Autodesk Inventor part; units mm, degrees
(part 2 of 2)
sketch "Náčrt39" plane through (0, 0, 15.5) normal (0, -1, 0) x (1, 0, 0)
  line L0 (-46, 13.2) -> (-46, 26.7)
  line L1 (-33, 26.7) -> (-46, 26.7)
  line L2 (-33, 26.7) -> (-33, 13.2)
  line L3 (-46, 13.2) -> (-33, 13.2)
  line L4 (-21.25, 15.889) -> (-21.25, 29.639)
  line L5 (-11.5, 29.639) -> (-21.25, 29.639)
  line L6 (-11.5, 29.639) -> (-11.5, 30.839)
  line L7 (-8.5, 30.839) -> (-11.5, 30.839)
  line L8 (-8.5, 29.639) -> (-8.5, 30.839)
  line L9 (-8.5, 29.639) -> (-8.5, 15.889)
  line L10 (-8.5, 15.889) -> (-21.25, 15.889)
  line L11 (0, 30.082064) -> (0, 0)
  line L12 (0, 30.082064) -> (-2, 30.082064)
  line L13 (-2, 30.082064) -> (-2, 24.139)
  line L14 (-2, 24.139) -> (-4.75, 24.139)
  line L15 (-4.75, 24.139) -> (-4.75, 30.082064)
  line L16 (-4.75, 30.082064) -> (-22.45, 30.082064)
  line L17 (-22.45, 18.2) -> (-22.45, 30.082064)
  line L18 (-22.45, 18.2) -> (-32.2, 18.2)
  line L19 (-32.2, 27.9) -> (-32.2, 18.2)
  line L20 (-32.2, 27.9) -> (-46.8, 27.9)
  line L21 (-46.8, 27.9) -> (-46.8, 9.2)
  line L22 (-49.5, 9.2) -> (-46.8, 9.2)
  line L23 (-49.5, 0) -> (-49.5, 9.2)
  line L24 (-40.88345, 0) -> (-49.5, 0)
  line L25 (-40.88345, 0) -> (-40.88345, -5)
  line L26 (-36.02558, -5) -> (-40.88345, -5)
  line L27 (-36.02558, 0) -> (-36.02558, -5)
  line L28 (0, 0) -> (-36.02558, 0)
  line L29 (-2.5, 4.1) -> (-2.5, 14.689)
  line L30 (-2.5, 4.1) -> (-21.25, 4.1)
  line L31 (-21.25, 14.689) -> (-21.25, 4.1)
  line L32 (-2.5, 14.689) -> (-21.25, 14.689)
  line L33 (-46, 13.2) -> (-46, 26.7)
  line L34 (-46, 26.7) -> (-46, 27.9)
  line L35 (-32.2, 27.9) -> (-46.8, 27.9)
  line L36 (-45.6, 27.9) -> (-45.6, 21.7)
  line L37 (-45.6, 21.7) -> (-46, 21.7)
  line L38 (-33, 26.7) -> (-33, 27.9)
  line L39 (-33.4, 27.9) -> (-33.4, 21.7)
  line L40 (-33.4, 21.7) -> (-33, 21.7)
  line L41 (-21.25, 24.639) -> (-20.85, 24.639)
  line L42 (-20.85, 24.639) -> (-20.85, 30.839)
  line L43 (-21.25, 30.839) -> (-21.25, 29.639)
  line L44 (-8.9, 30.839) -> (-8.9, 24.639)
  line L45 (-8.9, 24.639) -> (-8.5, 24.639)
  line L46 (-8.5, 30.839) -> (-22.45, 30.839)
  point P0 (0, -15.5)
  point P1 (-21.45, 29.639)
  point P2 (-20.85, 29.639)
  point P3 (-21.45, 29.639)
  dimension "d1" = 2
  dimension "d347" = 0.4
  dimension "d348" = 5
  constraints: 22 end point, 13 point on line, 8 perpendicular, 5 equal length, 1 horizontal, 1 vertical
  measures "d347" distance between parallel lines of L0 L36
  measures "d348" distance between parallel lines of L37 L1
extrude "Vysunutí57" cut sketch "Náčrt39" against normal up to next contours L0 L1 L36 L37 | L34 L20 L36 L1 | L40 L39 L1 L2 | L1 L39 L20 L38 | L43 L46 L42 L16 | L16 L42 L5 L43 | L5 L42 L41 L4 | L44 L7 L8 L16 | L16 L8 L9 L45 L44
sketch "Náčrt40" plane through (-2.5, 0, 0) normal (-1, 0, 0) x (0, 0, 1)
  arc A0 (19.6, 15.5) -> (19.590814, 16.1) centre (0, 15.5) ccw
  arc A1 (19.590814, 16.1) -> (19.391686, 18.35) centre (0, 15.5) ccw
  arc A2 (19.391686, 18.35) -> (18.626594, 21.6) centre (0, 15.5) ccw
  arc A3 (18.626594, 21.6) -> (16.295147, 26.391657) centre (0, 15.5) ccw
  arc A4 (18.594508, 21.697118) -> (16.295147, 26.391657) centre (0, 15.5) ccw
  arc A5 (14.149289, 29.063098) -> (13.25, 29.942905) centre (0, 15.5) ccw
  arc A6 (13.25, 29.942905) -> (7.756288, 33.5) centre (0, 15.5) ccw
  arc A7 (19.6, 15.5) -> (7.756288, 33.5) centre (0, 15.5) ccw
  line L0 (7.193747, 33.5) -> (7.756288, 33.5)
  line L1 (13.25, 33.5) -> (7.756288, 33.5)
  line L2 (7.193747, 33.5) -> (13.25, 33.5)
  line L3 (7.193747, 33.5) -> (7.756288, 33.5)
  line L4 (7.193747, 33.5) -> (5.792097, 33.5)
  line L5 (5.792097, 33.5) -> (5.792097, 33.450985)
  line L6 (7.756288, 33.450985) -> (5.792097, 33.450985)
  line L7 (7.756288, 33.5) -> (7.756288, 33.450985)
  ellipse E0 centre (5.792097, 32.402567) end of major axis (6.890446, 32.402567) minor radius 1.097433 (5.792097, 33.5) -> (4.693747, 32.402567) ccw
  line L8 (4.693747, 32.402567) -> (4.693747, 32.353552)
  ellipse E1 centre (5.792097, 32.353552) end of major axis (6.890446, 32.353552) minor radius 1.097433 (5.792097, 33.450985) -> (4.693747, 32.353552) ccw
  line L9 (5.792097, 33.5) -> (5.792097, 33.450985)
  line L10 (4.693747, 32.402567) -> (4.693747, 29.75313)
  line L11 (4.693747, 29.75313) -> (4.693747, 29.704115)
  line L12 (4.693747, 32.353552) -> (4.693747, 29.704115)
  line L13 (4.693747, 32.402567) -> (4.693747, 32.353552)
  ellipse E2 centre (8.443747, 29.75313) end of major axis (12.193747, 29.75313) minor radius 3.74687 (4.693747, 29.75313) -> (6.568747, 26.508244) ccw
  line L14 (6.568747, 26.508244) -> (6.568747, 26.45923)
  ellipse E3 centre (8.443747, 29.704115) end of major axis (12.193747, 29.704115) minor radius 3.74687 (4.693747, 29.704115) -> (6.568747, 26.45923) ccw
  line L15 (4.693747, 29.75313) -> (4.693747, 29.704115)
  line L16 (6.568747, 26.508244) -> (15.5, 21.356087)
  line L17 (15.5, 21.356087) -> (15.5, 21.307072)
  line L18 (6.568747, 26.45923) -> (15.5, 21.307072)
  line L19 (6.568747, 26.508244) -> (6.568747, 26.45923)
  line L20 (5.193747, 28.839806) -> (5.193747, 32.353552)
  arc A8 (5.590195, 32.75) -> (5.193747, 32.353552) centre (5.590195, 32.353552) ccw
  line L21 (5.590195, 32.75) -> (9.305778, 32.75)
  arc A9 (5.193747, 28.839806) -> (6.568747, 26.45923) centre (7.942027, 28.839806) ccw
  point P0 (0, 0)
  point P1 (9.305778, 32.75)
  point P2 (7.756288, 33.5)
extrude "Vysunutí58" cut sketch "Náčrt40" along normal through all contours L21 A8 L20 A9 E2 L11 L10 L8 E1 L6 L7 A6 | L7 L6 L5 L4 L0 | L5 E1 E0 | A9 E3 E2
sketch "Náčrt41" plane through (0, 32, 7.193747) normal (0, 0, -1) x (-1, 0, 0)
  line L0 (0, 1.5) -> (2.5, 1.5) projected
  line L1 (0, 1.5) -> (0, 3.5)
  line L2 (0, 3.5) -> (1, 3.5)
  line L3 (1, 3.5) -> (1, 2)
  line L4 (1, 2) -> (2, 2)
  line L5 (2, 2) -> (2, 1.5)
  line L6 (2, 2) -> (2.5, 1.5)
  point P0 (0, -32)
  dimension "d357" = 1
  dimension "d358" = 0.5
  dimension "d359" = 2
  dimension "d360" = 1
  constraints: 12 end point, 3 perpendicular, 1 horizontal, 1 point on line, 1 vertical
  measures "d357" distance of L1.end L2.end
  measures "d358" distance from line of L3.end L0
  measures "d359" distance between parallel lines of L0 L2
  measures "d360" distance of L3.end L4.end
extrude "Vysunutí59" add sketch "Náčrt41" against normal up to surface (6.056253 mm away)
sketch "Náčrt42" plane through (-46.8, 2.241154, 16.5) normal (-1, 0, 0) x (0, 0, 1)
  line L0 (20.7, -1.041154) -> (12.2, -1.041154)
  line L1 (12.2, -1.041154) -> (20.7, -1.041154)
  line L2 (20.7, -1.041154) -> (25.7, -1.041154)
  line L3 (25.7, -1.041154) -> (20.7, -1.041154)
  line L4 (26.9, 0.158846) -> (26.9, -2.241154)
  line L5 (26.9, -2.241154) -> (8.2, -2.241154)
  line L6 (25.7, -1.041154) -> (26.9, -1.041154)
  line L7 (18.9, -1.041154) -> (18.9, -2.241154)
  point P0 (-16.5, -2.241154)
  point P1 (18.9, -1.041154)
  dimension "d363" = 8
  constraints: 4 end point, 2 point on line, 1 midpoint, 1 perpendicular
  measures "d363" distance between parallel lines of L4 L7
extrude "Vysunutí60" add sketch "Náčrt42" along normal up to surface (2.7 mm away)
sketch "Náčrt43" plane through (-21.25, 0, 19.6) normal (1, 0, 0) x (0, 0, -1)
  arc A0 (10.294222, 32.75) -> (0, 15.5) centre (19.6, 15.5) ccw
  arc A1 (0.009186, 16.1) -> (0, 15.5) centre (19.6, 15.5) ccw
  arc A2 (0.208314, 18.35) -> (0.009186, 16.1) centre (19.6, 15.5) ccw
  arc A3 (0.973406, 21.6) -> (0.208314, 18.35) centre (19.6, 15.5) ccw
  arc A4 (3.304853, 26.391657) -> (0.973406, 21.6) centre (19.6, 15.5) ccw
  arc A5 (3.304853, 26.391657) -> (1.005492, 21.697118) centre (19.6, 15.5) ccw
  arc A6 (6.35, 29.942905) -> (5.450711, 29.063098) centre (19.6, 15.5) ccw
  arc A7 (10.294222, 32.75) -> (6.35, 29.942905) centre (19.6, 15.5) ccw
  line L0 (0, 8.6) -> (0, 15.5)
  line L1 (0, 15.5) -> (0, 15.450985)
  line L2 (0, 15.4) -> (0, 15.450985)
  line L3 (0, 15.4) -> (0, 0)
  line L4 (0, 2.75) -> (0, 0)
  line L5 (0, 2.75) -> (0, 8.6)
  line L6 (4.1, 15.4) -> (0, 15.4)
  line L7 (0, 15.4) -> (4.1, 15.4)
  line L8 (0, 15.4) -> (-5.4, 15.4)
  line L9 (0, 15.4) -> (-5.4, 15.4)
  line L10 (-3, 15.4) -> (0.255712, 18.655712)
  arc A8 (10.385659, 32.75) -> (0, 15.450985) centre (19.6, 15.450985) ccw
  line L11 (0.255712, 18.655712) -> (0.265376, 18.665376)
  point P0 (19.6, 0)
  point P1 (0, 15.5)
  dimension "d371" = 45
  dimension "d372" = 3
  constraints: 4 end point, 2 point on circle, 1 collinear, 1 point on line, 4 other
  measures "d371" angle of L9 L10
  measures "d372" distance of L10.start L2.start
extrude "Vysunutí61" add sketch "Náčrt43" against normal up to surface contours A0 L0 L8 L10 surface through (-27.984704, 23.450985, 12.146874) normal (-0.9991655, -0.0408458, 0)
sketch "Náčrt44" plane through (-33, 7.7, 33.7) normal (0, 0, 1) x (1, 0, 0)
  line L0 (6.412328, 10.955712) -> (11.75, 10.955712)
  ellipse E0 centre (556.934471, 30.3) end of major axis (1235.550967, 44.153501) minor radius 13.867971 (5.210931, 10.965376) -> (6.412328, 10.955712) ccw
  line L1 (5.210931, 10.965376) -> (5.344419, 7.7)
  line L2 (11.75, 7.7) -> (5.344419, 7.7)
  line L3 (11.75, 10.955712) -> (11.75, 7.7)
  line L4 (-12.2, 6.5) -> (10.55, 6.5)
  line L5 (10.55, 6.5) -> (10.55, 2.5)
  line L6 (10.55, 2.5) -> (11.75, 2.5)
  line L7 (11.75, 7.7) -> (11.75, 2.5)
  line L8 (-13.8, 7.7) -> (11.75, 7.7)
  line L9 (-13.8, 7.7) -> (-13.8, 2.5)
  line L10 (-12.2, 2.5) -> (-13.8, 2.5)
  line L11 (-12.2, 6.5) -> (-12.2, 2.5)
  line L12 (10.55, 2.5) -> (10.55, 0)
  line L13 (10.55, 0) -> (11.75, 0)
  line L14 (11.75, 2.5) -> (11.75, 0)
  line L15 (10.55, 2.5) -> (11.75, 2.5)
  line L16 (-13.8, 2.5) -> (-13.8, 0)
  line L17 (-12.2, 0) -> (-13.8, 0)
  line L18 (-12.2, 2.5) -> (-12.2, 0)
  line L19 (-12.2, 2.5) -> (-13.8, 2.5)
  line L20 (0, 0) -> (-13.8, 0)
  line L21 (0, 0) -> (11.75, 0)
  line L22 (0.8, -6.5) -> (0.8, 6.5)
  line L23 (0.8, 6.5) -> (0.8, 7.7)
  point P0 (33, -7.7)
  point P1 (5.344419, 7.7)
  point P2 (11.75, 2.5)
  point P3 (0.8, 0)
  constraints: 2 end point, 1 perpendicular, 1 point on line, 1 other
extrude "Vysunutí62" cut sketch "Náčrt44" against normal up to surface (14.1 mm away)
extrude "Vysunutí63" cut sketch "Náčrt44" against normal up to surface (16.2 mm away) contours L23 L4 L11 L10 L9 L8 | L22 L21 L20 L18 L11 L4 | L10 L18 L17 L16
extrude "Vysunutí64" cut sketch "Náčrt44" against normal up to surface contours L0 L3 L2 L1 E0 round surface about axis through (0, 15.5, 0) along (-1, 0, 0) radius 19.6 far side no
sketch "Náčrt23" plane through (-10.5, 28.878329, 20.540916) normal (0, 0.6427876, 0.7660444) x (1, 0, 0)
  line L0 (8, 6.236289) -> (8, 5.866304)
  line L1 (8, 6.236289) -> (-4.25, 6.236289)
  line L2 (-4.25, 4.25) -> (-4.25, 6.236289)
  line L3 (-4.25, 4.25) -> (0, 4.25)
  line L4 (0, 5.866304) -> (0, 4.25)
  line L5 (0, 5.866304) -> (8, 5.866304)
  line L6 (0, 5.866304) -> (0, 6.236289)
  line L7 (9.15, 4.779716) -> (9.15, 8.226916)
  line L8 (10.5, 8.226916) -> (9.15, 8.226916)
  line L9 (8, 5.866304) -> (8, 8.226916)
  line L10 (0, 5.866304) -> (8, 5.866304)
  line L11 (0, 5.866304) -> (0, 4.779716)
  line L12 (9.15, 4.779716) -> (0, 4.779716)
  line L13 (8, 5.866304) -> (8, 4.779716)
  line L14 (10.5, 9.759005) -> (10.5, 8.226916)
  line L15 (9.5, 9.759005) -> (10.5, 9.759005)
  line L16 (9.5, 8.609938) -> (9.5, 9.759005)
  line L17 (8.5, 8.609938) -> (9.5, 8.609938)
  line L18 (8, 8.226916) -> (8.5, 8.609938)
  point P0 (10.5, -8.918637)
  point P1 (8, 5.866304)
  point P2 (0, 4.779716)
  constraints: 4 end point, 2 perpendicular, 2 point on line
equation "\"d2\" = d1"
equation "\"d18\" = d17"
